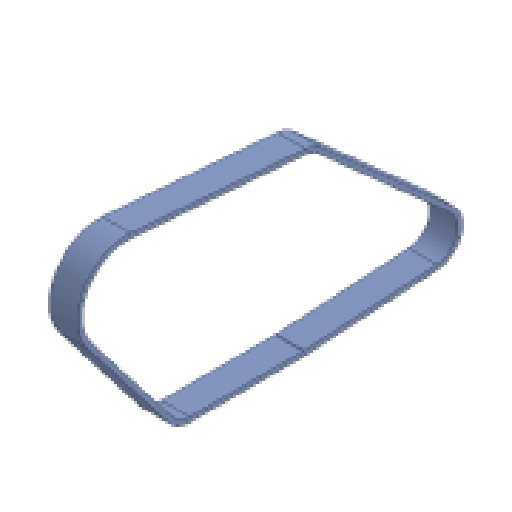
# Autodesk Inventor part: beltConifgV1
Saved by Autodesk Inventor 2025 (Build 290162000, 162)
## iProperties
Created: 2024-06-26
Part Number: beltConifgV1
Material: Generic
Document SubType Name: Modeling
Designer: derm
Density: 1 g/cm^3
Appearance: Rubber - Blue
Author: derm
Autodesk Inventor part; units mm, degrees
ref_plane "YZ Plane" through (0, 0, 0) normal (1, 0, 0) x (0, 1, 0)
ref_plane "XZ Plane" through (0, 0, 0) normal (0, 1, 0) x (-1, 0, 0)
ref_plane "XY Plane" through (0, 0, 0) normal (0, 0, 1) x (1, 0, 0)
sketch "Sketch1" plane through (0, 0, 0) normal (1, 0, 0) x (0, 1, 0)
  arc A0 (79.1037, -6.5576) -> (-48.559, 62.7887) centre (0, 0) ccw
  arc A1 (-235.3257, -81.6515) -> (-250.7337, -113.0458) centre (-211.0462, -113.0458) ccw
  arc A2 (-250.7337, -316.2458) -> (-250.6603, -318.6592) centre (-211.0462, -316.2458) ccw
  arc A3 (-236.1527, -556.7842) -> (-166.8315, -580.6877) centre (-196.5387, -554.3708) ccw
  arc A4 (43.2316, -343.563) -> (53.0762, -320.5249) centre (13.5244, -317.2461) ccw
  line L0 (-48.559, 62.7887) -> (-235.3257, -81.6515)
  line L1 (-250.7337, -113.0458) -> (-250.7337, -316.2458)
  line L2 (53.0762, -320.5249) -> (79.1037, -6.5576)
  line L3 (-250.6603, -318.6592) -> (-236.1527, -556.7842)
  line L4 (-166.8315, -580.6877) -> (43.2316, -343.563)
  line L5 (210.6942, -73.3583) -> (-226.1799, -73.3583) construction
  line L6 (206.7858, -594.0583) -> (-298.3784, -594.0583) construction
  line L7 (-211.0462, -113.0458) -> (-211.0462, -316.2458) construction
  line L8 (87.684, -7.2689) -> (61.6565, -321.2362)
  arc A5 (49.6762, -349.2721) -> (61.6565, -321.2362) centre (13.5244, -317.2461) ccw
  line L9 (49.6762, -349.2721) -> (-160.3869, -586.3968)
  arc A6 (-244.7465, -557.3078) -> (-160.3869, -586.3968) centre (-196.5387, -554.3708) ccw
  line L10 (-244.7465, -557.3078) -> (-259.2541, -319.1828)
  arc A7 (-259.3434, -316.2458) -> (-259.2541, -319.1828) centre (-211.0462, -316.2458) ccw
  line L11 (-259.3434, -316.2458) -> (-259.3434, -113.0458)
  arc A8 (-240.5928, -74.8408) -> (-259.3434, -113.0458) centre (-211.0462, -113.0458) ccw
  line L12 (-240.5928, -74.8408) -> (-53.8261, 69.5993)
  arc A9 (87.684, -7.2689) -> (-53.8261, 69.5993) centre (0, 0) ccw
  dimension "d0" = 158.75
  dimension "d1" = 79.375
  dimension "d2" = 79.375
  dimension "d3" = 79.375
  dimension "d4" = 79.375
  dimension "d6" = 520.7
  dimension "d7" = 203.2
  constraints: 26 end point, 20 point on circle, 12 tangent, 10 centre point, 2 horizontal, 1 coincident, 1 vertical, 9 other
  measures "d0" diameter of A0
  measures "d1" diameter of A1
  measures "d2" diameter of A2
  measures "d3" diameter of A3
  measures "d4" diameter of A4
  measures "d6" distance between parallel lines of L6 L5
  measures "d7" distance of L7.start L7.end
extrude "Extrusion1" add sketch "Sketch1" along normal blind 50.8
body "Solid1"
